Autodesk Inventor part; units mm, degrees
(part 2 of 2)
sketch "Sketch4" plane through (0, 0, 0) normal (0, -1, 0) x (1, 0, 0)
  circle A0 centre (-2.5088, -47.3592) radius 5
  arc A1 (-5.6088, -52.599) -> (-8.9192, -49.4269) centre (-8.7838, -52.599) ccw projected
  arc A2 (3.9015, -49.4269) -> (0.5912, -52.599) centre (3.7662, -52.599) ccw projected
  arc A3 (3.9015, -49.4269) -> (0.5912, -52.599) centre (3.7662, -52.599) ccw projected
  line L0 (0.5912, -52.599) -> (0.5912, -52.7956) projected
  arc A4 (0.5912, -52.7956) -> (0.6316, -53.1956) centre (2.5912, -52.7956) ccw projected
  line L1 (0.6316, -53.1956) -> (-5.6492, -53.1956) projected
  arc A5 (-5.6492, -53.1956) -> (-5.6088, -52.7956) centre (-7.6088, -52.7956) ccw projected
  line L2 (-5.6088, -52.7956) -> (-5.6088, -52.599) projected
  arc A6 (-5.6088, -52.599) -> (-8.9192, -49.4269) centre (-8.7838, -52.599) ccw projected
  arc A7 (-13.7066, -48.6137) -> (-8.9192, -49.4269) centre (-9.4136, -37.8395) ccw projected
  arc A8 (-13.7066, -48.6137) -> (-17.4405, -50.507) centre (-14.7393, -51.2055) ccw projected
  arc A9 (-20.0553, -52.5972) -> (-17.4405, -50.507) centre (-20.1417, -49.8085) ccw projected
  line L3 (-20.0553, -52.5972) -> (-36.2422, -37.6483) projected
  arc A10 (-36.2422, -37.6483) -> (-36.6182, -37.3815) centre (-37.4628, -38.97) ccw projected
  line L4 (-36.6182, -37.3815) -> (-55.6053, -27.2859) projected
  arc A11 (-55.6995, -27.0415) -> (-55.6053, -27.2859) centre (-55.5114, -27.1093) ccw projected
  line L5 (-55.6995, -27.0415) -> (-48.5506, -7.2175) projected
  arc A12 (-48.5506, -7.2175) -> (-49.5987, -4.9266) centre (-50.2437, -6.6069) ccw projected
  line L6 (-49.5987, -4.9266) -> (-52.1383, -3.9517) projected
  line L7 (-52.1383, -3.9517) -> (-52.0923, -3.8318) projected
  arc A13 (-52.0923, -3.8318) -> (-53.2165, -1.4748) centre (-53.7728, -3.1867) ccw projected
  line L8 (-53.2165, -1.4748) -> (-68.942, 3.6347) projected
  arc A14 (-69.0703, 3.8865) -> (-68.942, 3.6347) centre (-68.8803, 3.8248) ccw projected
  line L9 (-69.0703, 3.8865) -> (-68.2977, 6.2644) projected
  arc A15 (-68.2977, 6.2644) -> (-69.4534, 8.5324) centre (-70.0096, 6.8206) ccw projected
  line L10 (-69.4534, 8.5324) -> (-77.4605, 11.1341) projected
  arc A16 (-77.4605, 11.1341) -> (-78.6892, 11.0919) centre (-78.0168, 9.4221) ccw projected
  arc A17 (-79.0436, 11.5395) -> (-78.6892, 11.0919) centre (-76.4057, 13.2639) ccw projected
  arc A18 (-79.0436, 11.5395) -> (-84.7256, 10.6308) centre (-81.6815, 9.8151) ccw projected
  arc A19 (-86.3516, 8.632) -> (-84.7256, 10.6308) centre (-87.7697, 11.4464) ccw projected
  line L11 (-86.3516, 8.632) -> (-96.1954, 11.2696) projected
  arc A20 (-96.1954, 11.2696) -> (-98.4339, 9.8436) centre (-96.6613, 9.531) ccw projected
  line L12 (-98.4339, 9.8436) -> (-100.0229, 0.8316) projected
  arc A21 (-100.2546, 0.6694) -> (-100.0229, 0.8316) centre (-100.2199, 0.8664) ccw projected
  line L13 (-100.2546, 0.6694) -> (-124.8748, 5.0106) projected
  arc A22 (-125.0371, 5.2423) -> (-124.8748, 5.0106) centre (-124.8401, 5.2075) ccw projected
  line L14 (-125.0371, 5.2423) -> (-124.58, 7.8345) projected
  arc A23 (-124.58, 7.8345) -> (-126.1332, 9.9335) centre (-126.3526, 8.147) ccw projected
  line L15 (-126.1332, 9.9335) -> (-142.685, 11.9658) projected
  arc A24 (-142.8593, 12.1889) -> (-142.685, 11.9658) centre (-142.6606, 12.1645) ccw projected
  line L16 (-142.8593, 12.1889) -> (-141.1064, 26.4648) projected
  arc A25 (-139.1875, 26.9825) -> (-141.1064, 26.4648) centre (-139.5094, 24.3607) ccw projected
  arc A26 (-139.1875, 26.9825) -> (-138.5437, 32.2262) centre (-138.8656, 29.6043) ccw projected
  arc A27 (-140.2803, 33.1927) -> (-138.5437, 32.2262) centre (-138.2217, 34.848) ccw projected
  line L17 (-140.2803, 33.1927) -> (-138.5451, 47.3249) projected
  arc A28 (-138.3222, 47.499) -> (-138.5451, 47.3249) centre (-138.3466, 47.3005) ccw projected
  line L18 (-138.3222, 47.499) -> (-119.7209, 45.2151) projected
  arc A29 (-119.7209, 45.2151) -> (-117.7289, 46.6891) centre (-119.5015, 47.0016) ccw projected
  line L19 (-117.7289, 46.6891) -> (-115.938, 56.8462) projected
  arc A30 (-115.7062, 57.0084) -> (-115.938, 56.8462) centre (-115.7409, 56.8114) ccw projected
  line L20 (-115.7062, 57.0084) -> (-96.0551, 53.5435) projected
  arc A31 (-96.0551, 53.5435) -> (-94.0039, 54.8502) centre (-95.7426, 55.3161) ccw projected
  line L21 (-94.0039, 54.8502) -> (-91.432, 64.4488) projected
  arc A32 (-91.187, 64.5902) -> (-91.432, 64.4488) centre (-91.2388, 64.397) ccw projected
  line L22 (-91.187, 64.5902) -> (-72.7252, 59.6434) projected
  arc A33 (-72.7252, 59.6434) -> (-71.9812, 59.6037) centre (-72.2593, 61.3821) ccw projected
  arc A34 (-71.6418, 59.1189) -> (-71.9812, 59.6037) centre (-74.695, 57.3423) ccw projected
  arc A35 (-71.6418, 59.1189) -> (-65.229, 59.8039) centre (-68.5886, 60.8955) ccw projected
  arc A36 (-63.1542, 62.0029) -> (-65.229, 59.8039) centre (-61.8694, 58.7123) ccw projected
  line L23 (-63.1542, 62.0029) -> (-45.529, 56.2761) projected
  arc A37 (-45.4005, 56.024) -> (-45.529, 56.2761) centre (-45.5908, 56.0858) ccw projected
  line L24 (-45.4005, 56.024) -> (-46.1731, 53.6464) projected
  arc A38 (-46.1731, 53.6464) -> (-45.0175, 51.3783) centre (-44.4612, 53.0901) ccw projected
  line L25 (-45.0175, 51.3783) -> (-28.8495, 46.1251) projected
  arc A39 (-28.721, 45.8729) -> (-28.8495, 46.1251) centre (-28.9113, 45.9348) ccw projected
  line L26 (-28.721, 45.8729) -> (-28.8453, 45.4905) projected
  arc A40 (-28.8453, 45.4905) -> (-27.7784, 43.2539) centre (-27.1334, 44.9343) ccw projected
  line L27 (-27.7784, 43.2539) -> (-15.1483, 38.4057) projected
  arc A41 (-15.0076, 35.8329) -> (-15.1483, 38.4057) centre (-17.9498, 36.9623) ccw projected
  arc A42 (-15.0076, 35.8329) -> (-13.0469, 31.7087) centre (-12.0655, 34.7035) ccw projected
  arc A43 (-11.6856, 30.5543) -> (-13.0469, 31.7087) centre (-13.784, 29.4597) ccw projected
  line L28 (-11.6856, 30.5543) -> (-12.3214, 28.8982) projected
  arc A44 (-12.3214, 28.8982) -> (-10.641, 26.4532) centre (-10.641, 28.2531) ccw projected
  line L29 (-10.641, 26.4532) -> (5.6231, 26.4532) projected
  arc A45 (5.6231, 26.4532) -> (7.3035, 28.8983) centre (5.623, 28.2533) ccw projected
  line L30 (7.3035, 28.8983) -> (6.6678, 30.5543) projected
  arc A46 (8.0291, 31.7087) -> (6.6678, 30.5543) centre (8.7661, 29.4597) ccw projected
  arc A47 (8.0291, 31.7087) -> (9.9898, 35.8329) centre (7.0476, 34.7035) ccw projected
  arc A48 (10.1305, 38.4057) -> (9.9898, 35.8329) centre (12.932, 36.9623) ccw projected
  line L31 (10.1305, 38.4057) -> (22.7606, 43.2539) projected
  arc A49 (22.7606, 43.2539) -> (23.8274, 45.4906) centre (22.1155, 44.9344) ccw projected
  line L32 (23.8274, 45.4906) -> (23.7031, 45.8731) projected
  arc A50 (23.8315, 46.1251) -> (23.7031, 45.8731) centre (23.8933, 45.9349) ccw projected
  line L33 (23.8315, 46.1251) -> (39.9995, 51.3784) projected
  arc A51 (39.9995, 51.3784) -> (41.1552, 53.6465) centre (39.4433, 53.0903) ccw projected
  line L34 (41.1552, 53.6465) -> (40.3826, 56.0242) projected
  arc A52 (40.511, 56.2762) -> (40.3826, 56.0242) centre (40.5728, 56.086) ccw projected
  line L35 (40.511, 56.2762) -> (58.1363, 62.003) projected
  arc A53 (60.2111, 59.804) -> (58.1363, 62.003) centre (56.8515, 58.7124) ccw projected
  arc A54 (60.2111, 59.804) -> (66.6239, 59.119) centre (63.5707, 60.8956) ccw projected
  arc A55 (66.9633, 59.6038) -> (66.6239, 59.119) centre (69.6771, 57.3425) ccw projected
  arc A56 (66.9633, 59.6038) -> (67.7074, 59.6435) centre (67.2415, 61.3823) ccw projected
  line L36 (67.7074, 59.6435) -> (86.1692, 64.5904) projected
  arc A57 (86.4141, 64.449) -> (86.1692, 64.5904) centre (86.2209, 64.3972) ccw projected
  line L37 (86.4141, 64.449) -> (88.9861, 54.8504) projected
  arc A58 (88.9861, 54.8504) -> (91.0373, 53.5436) centre (90.7247, 55.3162) ccw projected
  line L38 (91.0373, 53.5436) -> (110.6885, 57.0087) projected
  arc A59 (110.9201, 56.8465) -> (110.6885, 57.0087) centre (110.7232, 56.8118) ccw projected
  line L39 (110.9201, 56.8465) -> (112.711, 46.6893) projected
  arc A60 (112.711, 46.6893) -> (114.7031, 45.2153) centre (114.4838, 47.0019) ccw projected
  line L40 (114.7031, 45.2153) -> (133.3044, 47.4992) projected
  arc A61 (133.5273, 47.3251) -> (133.3044, 47.4992) centre (133.3287, 47.3007) ccw projected
  line L41 (133.5273, 47.3251) -> (135.2625, 33.193) projected
  arc A62 (133.5258, 32.2264) -> (135.2625, 33.193) centre (133.2039, 34.8482) ccw projected
  arc A63 (133.5258, 32.2264) -> (134.1697, 26.9828) centre (133.8477, 29.6046) ccw projected
  arc A64 (136.0886, 26.465) -> (134.1697, 26.9828) centre (134.4916, 24.3609) ccw projected
  line L42 (136.0886, 26.465) -> (137.8415, 12.1889) projected
  arc A65 (137.6674, 11.9661) -> (137.8415, 12.1889) centre (137.6431, 12.1645) ccw projected
  line L43 (137.6674, 11.9661) -> (121.1155, 9.9338) projected
  arc A66 (121.1155, 9.9338) -> (119.5622, 7.8346) centre (121.3349, 8.1472) ccw projected
  line L44 (119.5622, 7.8346) -> (120.0193, 5.2424) projected
  arc A67 (119.8571, 5.0108) -> (120.0193, 5.2424) centre (119.8224, 5.2077) ccw projected
  line L45 (119.8571, 5.0108) -> (95.2368, 0.6696) projected
  arc A68 (95.0052, 0.8317) -> (95.2368, 0.6696) centre (95.2021, 0.8665) ccw projected
  line L46 (95.0052, 0.8317) -> (93.4161, 9.8437) projected
  arc A69 (93.4161, 9.8437) -> (91.1776, 11.2698) centre (91.6435, 9.5312) ccw projected
  line L47 (91.1776, 11.2698) -> (81.3338, 8.6321) projected
  arc A70 (79.7078, 10.6309) -> (81.3338, 8.6321) centre (82.7519, 11.4465) ccw projected
  arc A71 (79.7078, 10.6309) -> (74.0258, 11.5396) centre (76.6637, 9.8152) ccw projected
  arc A72 (73.6714, 11.092) -> (74.0258, 11.5396) centre (71.388, 13.264) ccw projected
  arc A73 (73.6714, 11.092) -> (72.4427, 11.1342) centre (72.999, 9.4222) ccw projected
  line L48 (72.4427, 11.1342) -> (64.4357, 8.5325) projected
  arc A74 (64.4357, 8.5325) -> (63.28, 6.2643) centre (64.9919, 6.8206) ccw projected
  line L49 (63.28, 6.2643) -> (64.0525, 3.8869) projected
  arc A75 (63.924, 3.6347) -> (64.0525, 3.8869) centre (63.8622, 3.825) ccw projected
  line L50 (63.924, 3.6347) -> (46.3947, -2.0609) projected
  line L51 (46.3947, -2.0609) -> (47.0489, -3.7648) projected
  arc A76 (46.9338, -4.0233) -> (47.0489, -3.7648) centre (46.8621, -3.8365) ccw projected
  line L52 (46.9338, -4.0233) -> (44.5811, -4.9264) projected
  arc A77 (44.5811, -4.9264) -> (43.5328, -7.2176) centre (45.2262, -6.6069) ccw projected
  line L53 (43.5328, -7.2176) -> (50.6818, -27.0414) projected
  arc A78 (50.5875, -27.2858) -> (50.6818, -27.0414) centre (50.4936, -27.1092) ccw projected
  line L54 (50.5875, -27.2858) -> (31.6006, -37.3813) projected
  arc A79 (31.6006, -37.3813) -> (31.2243, -37.6484) centre (32.4462, -38.9715) ccw projected
  line L55 (31.2243, -37.6484) -> (15.0376, -52.5972) projected
  arc A80 (12.4228, -50.507) -> (15.0376, -52.5972) centre (15.124, -49.8084) ccw projected
  arc A81 (12.4228, -50.507) -> (8.6889, -48.6136) centre (9.7216, -51.2055) ccw projected
  arc A82 (3.9015, -49.4269) -> (8.6889, -48.6136) centre (4.3959, -37.8394) ccw projected
  arc A83 (89.7588, 55.0574) -> (90.8984, 54.3314) centre (90.7247, 55.3162) ccw projected
  line L56 (87.1869, 64.656) -> (89.7588, 55.0574) projected
  arc A84 (87.1869, 64.656) -> (85.9621, 65.3631) centre (86.2209, 64.3972) ccw projected
  line L57 (67.5003, 60.4163) -> (85.9621, 65.3631) projected
  arc A85 (66.2904, 61.0732) -> (67.5003, 60.4163) centre (67.2415, 61.3823) ccw projected
  line L58 (65.3003, 64.1204) -> (66.2904, 61.0732) projected
  arc A86 (65.3003, 64.1204) -> (64.0403, 64.7624) centre (64.3492, 63.8113) ccw projected
  line L59 (40.2638, 57.037) -> (64.0403, 64.7624) projected
  arc A87 (40.2638, 57.037) -> (39.6218, 55.7769) centre (40.5728, 56.086) ccw projected
  line L60 (40.3944, 53.3993) -> (39.6218, 55.7769) projected
  arc A88 (39.7523, 52.1392) -> (40.3944, 53.3993) centre (39.4433, 53.0903) ccw projected
  line L61 (23.5844, 46.8859) -> (39.7523, 52.1392) projected
  arc A89 (23.5844, 46.8859) -> (22.9423, 45.6258) centre (23.8933, 45.9349) ccw projected
  line L62 (23.0666, 45.2434) -> (22.9423, 45.6258) projected
  arc A90 (22.4739, 44.0008) -> (23.0666, 45.2434) centre (22.1155, 44.9344) ccw projected
  line L63 (4.3858, 37.0574) -> (22.4739, 44.0008) projected
  arc A91 (4.3858, 37.0574) -> (3.8105, 35.7654) centre (4.744, 36.1239) ccw projected
  line L64 (6.5567, 28.6116) -> (3.8105, 35.7654) projected
  arc A92 (5.6231, 27.2532) -> (6.5567, 28.6116) centre (5.623, 28.2533) ccw projected
  line L65 (-10.6409, 27.2532) -> (5.6231, 27.2532) projected
  arc A93 (-11.5745, 28.6116) -> (-10.6409, 27.2532) centre (-10.641, 28.2531) ccw projected
  line L66 (-8.8284, 35.7654) -> (-11.5745, 28.6116) projected
  arc A94 (-8.8284, 35.7654) -> (-9.4036, 37.0574) centre (-9.762, 36.1238) ccw projected
  line L67 (-27.4917, 44.0008) -> (-9.4036, 37.0574) projected
  arc A95 (-28.0844, 45.2433) -> (-27.4917, 44.0008) centre (-27.1334, 44.9343) ccw projected
  line L68 (-27.9602, 45.6258) -> (-28.0844, 45.2433) projected
  arc A96 (-27.9602, 45.6258) -> (-28.6022, 46.8859) centre (-28.9113, 45.9348) ccw projected
  line L69 (-44.7702, 52.1391) -> (-28.6022, 46.8859) projected
  arc A97 (-45.4122, 53.3992) -> (-44.7702, 52.1391) centre (-44.4612, 53.0901) ccw projected
  line L70 (-44.6397, 55.7769) -> (-45.4122, 53.3992) projected
  arc A98 (-44.6397, 55.7769) -> (-45.2817, 57.0369) centre (-45.5908, 56.0858) ccw projected
  line L71 (-69.0581, 64.7623) -> (-45.2817, 57.0369) projected
  arc A99 (-69.0581, 64.7623) -> (-70.3182, 64.1203) centre (-69.3671, 63.8112) ccw projected
  line L72 (-71.3083, 61.0731) -> (-70.3182, 64.1203) projected
  arc A100 (-72.5182, 60.4162) -> (-71.3083, 61.0731) centre (-72.2593, 61.3821) ccw projected
  line L73 (-90.98, 65.363) -> (-72.5182, 60.4162) projected
  arc A101 (-90.98, 65.363) -> (-92.2048, 64.6558) centre (-91.2388, 64.397) ccw projected
  line L74 (-94.7767, 55.0573) -> (-92.2048, 64.6558) projected
  arc A102 (-95.9163, 54.3313) -> (-94.7767, 55.0573) centre (-95.7426, 55.3161) ccw projected
  line L75 (-115.5673, 57.7963) -> (-95.9163, 54.3313) projected
  arc A103 (-115.5673, 57.7963) -> (-116.7258, 56.9851) centre (-115.7409, 56.8114) ccw projected
  line L76 (-118.5167, 46.828) -> (-116.7258, 56.9851) projected
  arc A104 (-119.6234, 46.0091) -> (-118.5167, 46.828) centre (-119.5015, 47.0016) ccw projected
  line L77 (-138.2247, 48.2931) -> (-119.6234, 46.0091) projected
  arc A105 (-138.2247, 48.2931) -> (-139.3392, 47.4224) centre (-138.3466, 47.3005) ccw projected
  line L78 (-143.6533, 12.2863) -> (-139.3392, 47.4224) projected
  arc A106 (-143.6533, 12.2863) -> (-142.7826, 11.1718) centre (-142.6606, 12.1645) ccw projected
  line L79 (-126.2308, 9.1395) -> (-142.7826, 11.1718) projected
  arc A107 (-125.3678, 7.9733) -> (-126.2308, 9.1395) centre (-126.3526, 8.147) ccw projected
  line L80 (-125.8249, 5.3812) -> (-125.3678, 7.9733) projected
  arc A108 (-125.8249, 5.3812) -> (-125.0138, 4.2228) centre (-124.8401, 5.2075) ccw projected
  line L81 (-100.3935, -0.1185) -> (-125.0138, 4.2228) projected
  arc A109 (-100.3935, -0.1185) -> (-99.2351, 0.6927) centre (-100.2199, 0.8664) ccw projected
  line L82 (-97.6461, 9.7046) -> (-99.2351, 0.6927) projected
  arc A110 (-96.4024, 10.4969) -> (-97.6461, 9.7046) centre (-96.6613, 9.531) ccw projected
  line L83 (-80.9116, 6.3461) -> (-96.4024, 10.4969) projected
  arc A111 (-80.9116, 6.3461) -> (-79.6868, 7.0532) centre (-80.6528, 7.3122) ccw projected
  line L84 (-78.9827, 9.681) -> (-79.6868, 7.0532) projected
  arc A112 (-77.7078, 10.3732) -> (-78.9827, 9.681) centre (-78.0168, 9.4221) ccw projected
  line L85 (-69.7006, 7.7716) -> (-77.7078, 10.3732) projected
  arc A113 (-69.0586, 6.5115) -> (-69.7006, 7.7716) centre (-70.0096, 6.8206) ccw projected
  line L86 (-69.8311, 4.1339) -> (-69.0586, 6.5115) projected
  arc A114 (-69.8311, 4.1339) -> (-69.1891, 2.8738) centre (-68.8803, 3.8248) ccw projected
  line L87 (-53.4637, -2.2357) -> (-69.1891, 2.8738) projected
  arc A115 (-52.8392, -3.5451) -> (-53.4637, -2.2357) centre (-53.7728, -3.1867) ccw projected
  line L88 (-53.1719, -4.4119) -> (-52.8392, -3.5451) projected
  line L89 (-49.8855, -5.6734) -> (-53.1719, -4.4119) projected
  arc A116 (-49.3032, -6.9462) -> (-49.8855, -5.6734) centre (-50.2437, -6.6069) ccw projected
  line L90 (-56.4521, -26.7701) -> (-49.3032, -6.9462) projected
  arc A117 (-56.4521, -26.7701) -> (-55.9808, -27.9922) centre (-55.5114, -27.1093) ccw projected
  line L91 (-36.9938, -38.0878) -> (-55.9808, -27.9922) projected
  arc A118 (-36.7848, -38.2361) -> (-36.9938, -38.0878) centre (-37.4628, -38.97) ccw projected
  line L92 (-20.0076, -53.7302) -> (-36.7848, -38.2361) projected
  arc A119 (-20.0076, -53.7302) -> (-19.3291, -53.9956) centre (-19.3291, -52.9954) ccw projected
  line L93 (14.3114, -53.9956) -> (-19.3291, -53.9956) projected
  arc A120 (14.3114, -53.9956) -> (14.9899, -53.7302) centre (14.3114, -52.9955) ccw projected
  line L94 (31.7671, -38.236) -> (14.9899, -53.7302) projected
  arc A121 (31.9761, -38.0877) -> (31.7671, -38.236) centre (32.4462, -38.9715) ccw projected
  line L95 (50.9631, -27.9922) -> (31.9761, -38.0877) projected
  arc A122 (50.9631, -27.9922) -> (51.4343, -26.77) centre (50.4936, -27.1092) ccw projected
  line L96 (44.2854, -6.9461) -> (51.4343, -26.77) projected
  arc A123 (44.8677, -5.6733) -> (44.2854, -6.9461) centre (45.2262, -6.6069) ccw projected
  line L97 (47.2205, -4.7701) -> (44.8677, -5.6733) projected
  arc A124 (47.2205, -4.7701) -> (47.7958, -3.4782) centre (46.8621, -3.8365) ccw projected
  line L98 (47.4437, -2.5612) -> (47.7958, -3.4782) projected
  line L99 (64.1713, 2.8739) -> (47.4437, -2.5612) projected
  arc A125 (64.1713, 2.8739) -> (64.8134, 4.134) centre (63.8622, 3.825) ccw projected
  line L100 (64.0408, 6.5116) -> (64.8134, 4.134) projected
  arc A126 (64.6829, 7.7717) -> (64.0408, 6.5116) centre (64.9919, 6.8206) ccw projected
  line L101 (72.69, 10.3734) -> (64.6829, 7.7717) projected
  arc A127 (73.9649, 9.6812) -> (72.69, 10.3734) centre (72.999, 9.4222) ccw projected
  line L102 (74.669, 7.0534) -> (73.9649, 9.6812) projected
  arc A128 (74.669, 7.0534) -> (75.8938, 6.3463) centre (75.635, 7.3122) ccw projected
  line L103 (91.3846, 10.4971) -> (75.8938, 6.3463) projected
  arc A129 (92.6283, 9.7048) -> (91.3846, 10.4971) centre (91.6435, 9.5312) ccw projected
  line L104 (94.2173, 0.6929) -> (92.6283, 9.7048) projected
  arc A130 (94.2173, 0.6929) -> (95.3758, -0.1183) centre (95.2021, 0.8665) ccw projected
  line L105 (119.996, 4.2229) -> (95.3758, -0.1183) projected
  arc A131 (119.996, 4.2229) -> (120.8071, 5.3814) centre (119.8224, 5.2077) ccw projected
  line L106 (120.3501, 7.9735) -> (120.8071, 5.3814) projected
  arc A132 (121.213, 9.1397) -> (120.3501, 7.9735) centre (121.3349, 8.1472) ccw projected
  line L107 (137.7648, 11.1721) -> (121.213, 9.1397) projected
  arc A133 (137.7648, 11.1721) -> (138.6355, 12.2865) centre (137.6431, 12.1645) ccw projected
  line L108 (134.3213, 47.4226) -> (138.6355, 12.2865) projected
  arc A134 (134.3213, 47.4226) -> (133.2069, 48.2933) centre (133.3287, 47.3007) ccw projected
  line L109 (114.6056, 46.0093) -> (133.2069, 48.2933) projected
  arc A135 (113.4989, 46.8282) -> (114.6056, 46.0093) centre (114.4838, 47.0019) ccw projected
  line L110 (111.7079, 56.9853) -> (113.4989, 46.8282) projected
  arc A136 (111.7079, 56.9853) -> (110.5495, 57.7965) centre (110.7232, 56.8118) ccw projected
  line L111 (90.8984, 54.3314) -> (110.5495, 57.7965) projected
  circle A137 centre (9.7216, -51.2055) radius 1.1 projected
  circle A138 centre (-138.8656, 29.6043) radius 1.1 projected
  circle A139 centre (76.6637, 9.8152) radius 1.1 projected
  circle A140 centre (-14.7393, -51.2055) radius 1.1 projected
  circle A141 centre (-68.5886, 60.8955) radius 1.1 projected
  circle A142 centre (63.5707, 60.8956) radius 1.1 projected
  circle A143 centre (-12.0655, 34.7035) radius 1.1 projected
  circle A144 centre (7.0476, 34.7035) radius 1.1 projected
  circle A145 centre (133.8477, 29.6046) radius 1.1 projected
  circle A146 centre (-81.6815, 9.8151) radius 1.1 projected
  circle A147 centre (-137.3116, 16.3436) radius 5
  circle A148 centre (132.2938, 16.3438) radius 5
  circle A149 centre (-89.9006, 48.7121) radius 5
  circle A150 centre (87.4673, 49.3472) radius 5
  line L112 (40.511, 56.2762) -> (58.1363, 62.003) projected
  arc A151 (-71.6418, 59.1189) -> (-65.229, 59.8039) centre (-68.5886, 60.8955) ccw projected
  line L113 (-63.1542, 62.0029) -> (-45.529, 56.2761) projected
  line L114 (-142.8593, 12.1889) -> (-141.1064, 26.4648) projected
  line L115 (-126.1332, 9.9335) -> (-142.685, 11.9658) projected
  line L116 (137.6674, 11.9661) -> (121.1155, 9.9338) projected
  arc A152 (-46.1731, 53.6464) -> (-45.0175, 51.3783) centre (-44.4612, 53.0901) ccw projected
  arc A153 (39.9995, 51.3784) -> (41.1552, 53.6465) centre (39.4433, 53.0903) ccw projected
  arc A154 (88.9861, 54.8504) -> (91.0373, 53.5436) centre (90.7247, 55.3162) ccw projected
  line L117 (110.6885, 57.0087) -> (91.0373, 53.5436) projected
  arc A155 (83.4472, 52.3203) -> (86.1517, 65.3948) centre (70.6503, 61.7844) ccw
  line L118 (88.9861, 54.8504) -> (86.4141, 64.449) projected
  arc A156 (95.1362, 54.2663) -> (92.3178, 48.1337) centre (110.0546, 43.6963) ccw
  arc A157 (-92.2048, 61.5649) -> (-88.0697, 53.3648) centre (-85.5452, 59.7805) ccw
  arc A158 (-94.7888, 47.6608) -> (-101.9794, 54.5881) centre (-103.5325, 45.7803) ccw
  line L119 (-96.0551, 53.5435) -> (-115.7062, 57.0084) projected
  line L120 (-91.432, 64.4488) -> (-94.0039, 54.8502) projected
  point P0 (0, 0)
  point P1 (44.695, 57.6356)
  point P2 (60.622, 58.9504)
  point P3 (132.9031, 11.3811)
  point P4 (137.2565, 16.9532)
  point P5 (-6.3468, -50.564)
  point P6 (-5.6088, -52.599)
  point P7 (0.5912, -52.599)
  point P8 (1.3291, -50.564)
  point P9 (-137.9209, 11.3809)
  point P10 (-142.2743, 16.953)
  point P11 (-65.6399, 58.9503)
  point P12 (-49.7129, 57.6355)
  point P13 (86.3209, 64.5704)
  point P14 (89.8625, 53.7362)
  point P15 (95.1362, 54.2663)
  dimension "d9" = 10
  dimension "d10" = 10
  dimension "d11" = 10
  dimension "d12" = 10
  dimension "d13" = 10
  dimension "d16" = 5.969
  dimension "d17" = 3.2574
  dimension "d19" = 6.604
  dimension "d20" = 5.842
  constraints: 13 point on circle, 13 tangent, 9 centre point, 3 point on line, 2 other
  measures "d9" diameter of A0
  measures "d10" diameter of A147
  measures "d11" diameter of A148
  measures "d12" diameter of A149
  measures "d13" diameter of A150
  measures "d16" vertical distance of A150.centre A58.centre
  measures "d17" horizontal distance of A150.centre A58.centre
  measures "d19" vertical distance of A31.centre A149.centre
  measures "d20" horizontal distance of A31.centre A149.centre
extrude "Extrusion4" add sketch "Sketch4" against normal blind 0.4 contours A0 | A0 A2 L0 A4 L1 A5 L2 A1 | L15 A24 L16 A147 | A147 | A148 L42 A65 L43 | A148 | L20 A31 L21 A157 A149 A158 | A156 A150 A58 L38 | A149 | A150 | A150 A155 A57 L37 A58 | A83 L111 A136 L110 A135 L109 A134 L108 A133 L107 A132 L106 A131 L105 A130 L104 A129 L103 A128 L102 A127 L101 A126 L100 A125 L99 L98 A124 L97 A123 L96 A122 L95 A121 L94 A120 L93 A119 L92 A118 L91 A117 L90 A116 L89 L88 A115 L87 A114 L86 A113 L85 A112 L84 A111 L83 A110 L82 A109 L81 A108 L80 A107 L79 A106 L78 A105 L77 A104 L76 A103 L75 A102 L74 A101 L73 A100 L72 A99 L71 A98 L70 A97 L69 A96 L68 A95 L67 A94 L66 A93 L65 A92 L64 A91 L63 A90 L62 A89 L61 A88 L60 A87 L59 A86 L58 A85 L57 A84 L56
fillet "Fillet2" radius 3.175 1 edges at (95.1362, 0.2, 54.2663)
body "Solid1"
